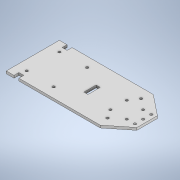
# Autodesk Inventor part: body
Saved by Autodesk Inventor 2022 (Build 260153000, 153)
## iProperties
Created: 2021-07-05
Part Number: body
Material: 一般
Document SubType Name: Modeling
Designer: ken
Density: 1 g/cm^3
Appearance: 既定
Author: ken
Autodesk Inventor part; units mm, degrees
ref_plane "YZ Plane" through (0, 0, 0) normal (1, 0, 0) x (0, 1, 0)
ref_plane "XZ Plane" through (0, 0, 0) normal (0, 1, 0) x (-1, 0, 0)
ref_plane "XY Plane" through (0, 0, 0) normal (0, 0, 1) x (1, 0, 0)
sketch "スケッチ1" plane through (0, 0, 0) normal (0, 1, 0) x (-1, 0, 0)
  line L0 (0, 0) -> (140, 0)
  line L1 (140, 0) -> (140, -65)
  line L2 (140, -65) -> (0, -65)
  line L3 (0, -65) -> (0, 0)
  line L4 (130.5, 0) -> (124.5, 0)
  line L5 (124.5, 0) -> (124.5, -6)
  line L6 (124.5, -6) -> (130.5, -6)
  line L7 (130.5, -6) -> (130.5, 0)
  line L8 (130.5, -65) -> (124.5, -65)
  line L9 (124.5, -65) -> (124.5, -59)
  line L10 (124.5, -59) -> (130.5, -59)
  line L11 (130.5, -59) -> (130.5, -65)
  line L12 (0, -45) -> (25, -65)
  line L13 (0, -20) -> (25, 0)
  line L14 (70, -25) -> (65, -25)
  line L15 (65, -25) -> (65, -40)
  line L16 (65, -40) -> (70, -40)
  line L17 (70, -40) -> (70, -25)
  point P0 (130.5, -3)
  point P1 (130.5, -62)
  dimension "d0" = 140
  dimension "d1" = 65
  dimension "d61" = 6
  dimension "d62" = 6
  dimension "d63" = 6
  dimension "d64" = 6
  dimension "d65" = 9.5
  dimension "d66" = 20
  dimension "d67" = 20
  dimension "d68" = 25
  dimension "d70" = 5
  dimension "d71" = 15
  dimension "d72" = 70
  dimension "d73" = 25
  constraints: 36 end point, 8 parallel, 6 point on line, 4 horizontal, 4 perpendicular, 2 midpoint, 2 vertical alignment
  measures "d0" distance of L1.end L2.end
  measures "d1" distance of L0.end L1.end
  measures "d61" distance of L6.end L5.end
  measures "d62" distance of L5.end L4.end
  measures "d63" distance of L9.end L10.end
  measures "d64" distance of L8.end L9.end
  measures "d65" distance from line of point (130.5, -3) L1
  measures "d66" distance of L0.start L13.start
  measures "d67" distance of L2.end L12.start
  measures "d68" distance of L0.start L13.end
  measures "d70" distance of L16.end L15.end
  measures "d71" distance of L15.end L14.end
  measures "d72" distance between parallel lines of L1 L17
  measures "d73" distance between parallel lines of L0 L14
extrude "押し出し1" add sketch "スケッチ1" along normal blind 3 contours L0 L5 L6 L7 L1 L2 L11 L10 L9 L12 L3 L13
sketch "スケッチ2" plane through (0, 3, 0) normal (0, 1, 0) x (1, 0, 0)
  line L0 (-140, 0) -> (0, 0) projected
  line L1 (-140, 65) -> (-140, 0) projected
  line L2 (-25, 65) -> (-140, 65) projected
  point P0 (-127.5, 12.5)
  point P1 (0, 65)
  point P2 (-127.5, 52.5)
  dimension "d9" = 12.5
  dimension "d12" = 12.5
  dimension "d55" = 12.5
  dimension "d69" = 40
  measures "d9" distance from line of L0 point (-127.5, 12.5)
  measures "d12" distance from line of point (-127.5, 12.5) L1
  measures "d55" distance from line of L2 point (-127.5, 52.5)
  measures "d69" distance of point (-127.5, 12.5) point (-127.5, 52.5)
hole "穴1" at (-127.5, 3, -12.5) at (-127.5, 3, -52.5) direction (0, -1, 0) diameter 3 end through all
sketch "スケッチ3" plane through (0, 3, 0) normal (0, 1, 0) x (1, 0, 0)
  line L0 (-140, 0) -> (0, 0) projected
  line L1 (-25, 65) -> (-140, 65) projected
  line L2 (0, 0) -> (0, 45) projected
  point P0 (-35, 22.5)
  point P1 (-35, 42.5)
  point P2 (-15, 42.5)
  point P3 (-15, 22.5)
  point P4 (0, 65)
  dimension "d20" = 20
  dimension "d21" = 20
  dimension "d22" = 22.5
  dimension "d24" = 15
  constraints: 2 horizontal alignment, 2 vertical alignment
  measures "d20" distance of point (-35, 42.5) point (-35, 22.5)
  measures "d21" distance of point (-15, 42.5) point (-35, 42.5)
  measures "d22" distance from line of L0 point (-35, 22.5)
  measures "d24" distance from line of L2 point (-15, 42.5)
hole "穴2" at (-35, 3, -22.5) at (-35, 3, -42.5) at (-15, 3, -42.5) at (-15, 3, -22.5) direction (0, -1, 0) diameter 3 end through all
sketch "スケッチ4" plane through (0, 3, 0) normal (0, 1, 0) x (1, 0, 0)
  line L0 (-25, 65) -> (-140, 65) projected
  line L1 (0, 0) -> (0, 45) projected
  point P0 (-5, 42.5)
  point P1 (-5, 32.5)
  point P2 (-5, 22.5)
  point P3 (0, 65)
  dimension "d32" = 10
  dimension "d33" = 10
  dimension "d34" = 32.5
  dimension "d35" = 5
  constraints: 2 vertical alignment
  measures "d32" distance of point (-5, 42.5) point (-5, 32.5)
  measures "d33" distance of point (-5, 22.5) point (-5, 32.5)
  measures "d34" distance from line of L0 point (-5, 32.5)
  measures "d35" distance from line of L1 point (-5, 42.5)
hole "穴3" at (-5, 3, -42.5) at (-5, 3, -32.5) at (-5, 3, -22.5) direction (0, -1, 0) diameter 3.2 end through all
sketch "スケッチ5" plane through (0, 3, 0) normal (0, 1, 0) x (1, 0, 0)
  line L0 (-25, 65) -> (-140, 65) projected
  line L1 (-140, 65) -> (-140, 0) projected
  point P0 (0, 0)
  point P1 (-94, 53)
  point P2 (-28, 53)
  point P3 (-28, 12)
  point P4 (-94, 12)
  point P5 (0, 65)
  dimension "d43" = 66
  dimension "d44" = 41
  dimension "d46" = 12
  dimension "d47" = 46
  constraints: 2 horizontal alignment, 2 vertical alignment
  measures "d43" distance of point (-94, 53) point (-28, 53)
  measures "d44" distance of point (-94, 12) point (-94, 53)
  measures "d46" distance from line of L0 point (-94, 53)
  measures "d47" distance from line of L1 point (-94, 53)
hole "穴4" at (-94, 3, -53) at (-28, 3, -53) at (-28, 3, -12) at (-94, 3, -12) direction (0, -1, 0) diameter 3.2 end through all
